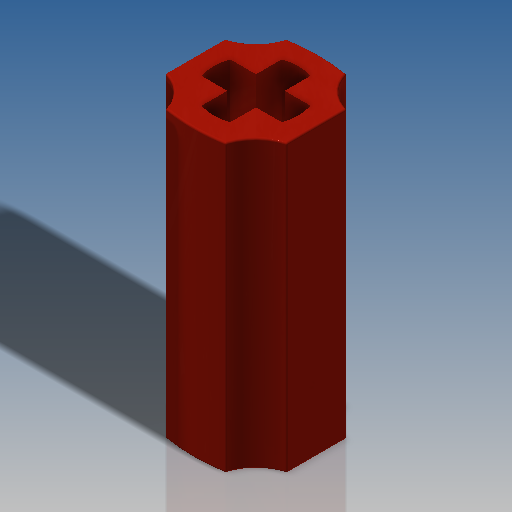
# Autodesk Inventor part: 6538c-Red
Saved by Autodesk Inventor 2018.3 (Build 223284000, 284)
## iProperties
Created: 2014-07-30
Part Number: 6538c-Red
Material: ABS Plastic
Document SubType Name: Modeling
Designer: D. Kohfeld
Mass: 0.445958 g
Surface Area: 7.28597 cm^2
Volume: 0.420715 cm^3
Density: 1.06 g/cm^3
Appearance: Red
Author: D. Kohfeld
Autodesk Inventor part; units mm, degrees
ref_plane "YZ Plane" through (0, 0, 0) normal (1, 0, 0) x (0, 1, 0)
ref_plane "XZ Plane" through (0, 0, 0) normal (0, 1, 0) x (-1, 0, 0)
ref_plane "XY Plane" through (0, 0, 0) normal (0, 0, 1) x (1, 0, 0)
sketch "Sketch2" plane through (0, 0, 0) normal (0, 1, 0) x (-1, 0, 0)
  circle A0 centre (0, 0) radius 3.52 construction
  circle A1 centre (0, 0) radius 2.3784 construction
  line L0 (-4, 4) -> (4, 4) construction
  line L1 (4, 4) -> (4, -4) construction
  line L2 (-0.8, 2.2399) -> (-0.8, 0.8)
  line L3 (-0.8, 0.8) -> (-2.2399, 0.8)
  line L4 (-2.2399, -0.8) -> (-0.8, -0.8)
  line L5 (-0.8, -0.8) -> (-0.8, -2.2399)
  line L6 (0.8, -2.2399) -> (0.8, -0.8)
  line L7 (0.8, -0.8) -> (2.2399, -0.8)
  line L8 (2.2399, 0.8) -> (0.8, 0.8)
  line L9 (0.8, 0.8) -> (0.8, 2.2399)
  arc A2 (0.8, 2.2399) -> (-0.8, 2.2399) centre (0, 0) ccw
  arc A3 (-2.2399, 0.8) -> (-2.2399, -0.8) centre (0, 0) ccw
  arc A4 (-0.8, -2.2399) -> (0.8, -2.2399) centre (0, 0) ccw
  arc A5 (2.2399, -0.8) -> (2.2399, 0.8) centre (0, 0) ccw
  circle A6 centre (-4, 4) radius 2.4
  circle A7 centre (4, 4) radius 2.4
  circle A8 centre (-4, -4) radius 2.4
  circle A9 centre (4, -4) radius 2.4
  arc A10 (1.6845, 3.3686) -> (-1.6845, 3.3686) centre (0, -5.93) ccw
  line L10 (-3.4, 1.6762) -> (-3.4, -1.6762)
  line L11 (3.4, 1.6762) -> (3.4, -1.6762)
  arc A11 (-1.6845, -3.3686) -> (1.6845, -3.3686) centre (0, 5.93) ccw
  circle A12 centre (0, 0) radius 1.1314
  point P0 (0, 4)
  point P1 (4, 0)
  dimension "d0" = 4.7569
  dimension "d1" = 7.04
  dimension "d2" = 8
  dimension "d4" = 1.6
  dimension "d20" = 4.8
  dimension "d21" = 18.9
  dimension "d22" = 6.8
  constraints: 24 end point, 20 point on circle, 11 centre point, 9 equal length, 6 coincident, 6 parallel, 4 equal radius, 4 horizontal alignment, 4 perpendicular, 2 midpoint, 2 tangent, 2 vertical alignment, 1 horizontal, 1 vertical, 17 other
  measures "d1" diameter of A0
  measures "d2" distance of L0.start L0.end
  measures "d4" distance between parallel lines of L9 L2
  measures "d20" diameter of A6
  measures "d21" diameter of A10
  measures "d22" distance between parallel lines of L10 L11
extrude "Extrusion1" add sketch "Sketch2" along normal mid plane 16 contours A6 A10 A7 L11 A9 A11 A8 L10
extrude "Extrusion3" add sketch "Sketch2" along normal mid plane 0.2 contours A2 L9 A12 L2 | A12 L4 A3 L3 | L8 A5 L7 A12 | A12 L6 A4 L5
fillet "Fillet1" radius 0.1 24 edges at (1.6845, 0, 3.3686) (3.4, 0, 1.6762) (-1.6845, 0, 3.3686) (-3.4, 0, 1.6762) (3.4, 0, -1.6762) (1.6845, 0, -3.3686) (-1.6845, 0, -3.3686) (-3.4, 0, -1.6762) (0, 8, 3.52) (-2.3145, 8, 2.2915) (-3.4, 8, 0) (-2.3145, 8, -2.2915) (0, 8, -3.52) (2.3145, 8, -2.2915) (3.4, 8, 0) (2.3145, 8, 2.2915) (2.3145, -8, 2.2915) (0, -8, 3.52) (-2.3145, -8, 2.2915) (-3.4, -8, 0) (-2.3145, -8, -2.2915) (0, -8, -3.52) (2.3145, -8, -2.2915) (3.4, -8, 0)
equation "\"d2\" = lu"
equation "\"d4\" = axlet"
equation "\"lu\" = 8"
equation "\"axlet\" = 1.6"
body "Solid1"
